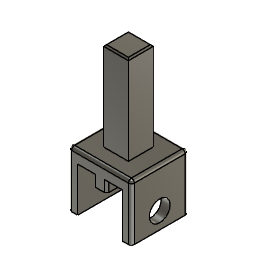
Slider (Autodesk Fusion 360 design; units mm, degrees)
Autodesk Fusion 360 part; units mm, degrees
sketch "Sketch1" plane through (0, 0, 0) normal (0, 1, 0) x (1, 0, 0)
  line L0 (0, 0) -> (6, 0)
  line L1 (6, 0) -> (6, -38)
  line L2 (6, -38) -> (0, -38)
  line L3 (0, -38) -> (0, 0)
  line L4 (0, -38) -> (42.4, -38)
  line L5 (42.4, -38) -> (42.4, -30)
  line L6 (42.4, -30) -> (0, -30)
  line L7 (0, -30) -> (0, -38)
  line L8 (42.4, -38) -> (36.4, -38)
  line L9 (36.4, -38) -> (36.4, 0)
  line L10 (36.4, 0) -> (42.4, 0)
  line L11 (42.4, 0) -> (42.4, -38)
  line L12 (16.75, -38) -> (25.65, -38)
  line L13 (25.65, -38) -> (25.65, -22.4)
  line L14 (25.65, -22.4) -> (16.75, -22.4)
  line L15 (16.75, -22.4) -> (16.75, -38)
  dimension "d1" = 6
  dimension "d2" = 38
  dimension "d3" = 8
  dimension "d5" = 6
  dimension "d6" = 38
  dimension "d8" = 15.6
  dimension "d9" = 10.75
  dimension "d29" = 10.75
  dimension "d30" = 42.4
  constraint horizontal L0
  constraint vertical L1
  constraint horizontal L2
  constraint vertical L3
  constraint coincident L0.start L3.end
  constraint horizontal L4
  constraint vertical L5
  constraint horizontal L6
  constraint vertical L7
  constraint horizontal L8
  constraint vertical L9
  constraint horizontal L10
  constraint vertical L11
  constraint horizontal L12
  constraint vertical L13
  constraint horizontal L14
  constraint vertical L15
  constraint coincident L4 L12.start
  measures "d1" distance of L0.start L0.end
  measures "d2" distance of L0.start L2.end
  measures "d3" distance of L2.end L6.end
  measures "d5" distance of L4.end L8.end
  measures "d6" distance of L4.end L10.end
  measures "d8" distance of L12.start L14.end L0.start
  measures "d9" distance of L1 L15 L0.start
  measures "d29" distance of L9 L13
  measures "d30" distance of L3 L11
extrude "Extrude1" add sketch "Sketch1" along normal blind 38.4
sketch "Sketch2" plane through (0, 0, 38) normal (0, 0, 1) x (-1, 0, 0)
  line L0 (0, 0) -> (-42.4, 0)
  line L1 (-42.4, 0) -> (-42.4, -38.4)
  line L2 (-42.4, -38.4) -> (0, -38.4)
  line L3 (0, -38.4) -> (0, 0)
  line L4 (-42.4, -38.4) -> (0, 0) construction
  line L5 (0, -38.4) -> (-42.4, 0) construction
  line L6 (-29.6, -10.8) -> (-12.8, -10.8)
  line L7 (-12.8, -10.8) -> (-12.8, -27.6)
  line L8 (-12.8, -27.6) -> (-29.6, -27.6)
  line L9 (-29.6, -27.6) -> (-29.6, -10.8)
  line L10 (-29.6, -10.8) -> (-12.8, -27.6) construction
  line L11 (-12.8, -10.8) -> (-29.6, -27.6) construction
  point P0 (-21.2, -19.2)
  dimension "d12" = 16.8
  dimension "d13" = 16.8
  constraint coincident L1.end L2.start
  constraint coincident L0.start L3.end
  constraint coincident L2.end L3.start
  constraint coincident L0.end L1.start
  constraint perpendicular L6 L7
  constraint parallel L6 L8
  constraint parallel L7 L9
  constraint horizontal L6
  constraint coincident L10 P0
  constraint coincident L11 P0
  constraint midpoint L4 P0
  measures "d12" distance of L6.end L7.end
  measures "d13" distance of L7.end L8.end
extrude "Extrude2" add sketch "Sketch2" along normal blind 60 contours L6 L7 L8 L9
chamfer "Chamfer1" distance 1 angle 45 4 edges at (21.2, 10.8, 98) (29.6, 19.2, 98) (12.8, 19.2, 98) (21.2, 27.6, 98)
sketch "Sketch3" plane through (0, 0, 0) normal (-1, 0, 0) x (0, -1, 0)
  line L0 (0, 0) -> (0, 38)
  line L1 (0, 38) -> (-38.4, 38)
  line L2 (-38.4, 38) -> (-38.4, 0)
  line L3 (-38.4, 0) -> (0, 0)
  line L4 (-38.4, 0) -> (0, 0)
  line L5 (0, 0) -> (0, 22.4)
  line L6 (0, 22.4) -> (-38.4, 22.4)
  line L7 (-38.4, 22.4) -> (-38.4, 0)
  line L8 (-38.4, 22.4) -> (0, 0) construction
  line L9 (0, 22.4) -> (-38.4, 0) construction
  circle A0 centre (-19.2, 11.2) radius 6
  dimension "d18" = 22.4
  dimension "d19" = 12
  constraint horizontal L4
  constraint vertical L5
  constraint horizontal L6
  constraint vertical L7
  constraint coincident L2.end L3.start
  constraint midpoint L9 A0.centre
  measures "d18" distance of L2.end L6.end
  measures "d19" diameter of A0
extrude "Extrude3" cut sketch "Sketch3" against normal up to surface (6 mm away) contours A0
sketch "Sketch4" plane through (42.4, 0, 0) normal (1, 0, 0) x (0, 1, 0)
  line L0 (0, 38) -> (0, 0)
  line L1 (0, 0) -> (38.4, 0)
  line L2 (38.4, 0) -> (38.4, 38)
  line L3 (38.4, 38) -> (0, 38)
  circle A0 centre (19.2, 11.2) radius 6
  circle A1 centre (19.2, 11.2) radius 7
  dimension "d22" = 1
extrude "Extrude4" cut sketch "Sketch4" against normal up to surface (6 mm away) contours A0 | A1
thread "Thread1" "ISO Metric profile 12.0 M12x1.75 6H" major diameter 12.2265 minor diameter 10.2735 pitch 1.75 angle 60 modelled right hand crest width 0.4769 on face at (4, 13.2075, 10.9009) crest through (0.4375, 14.0633, 11.2)
fillet "Fillet1" radius 2 8 edges at (21.2, 0, 38) (0, 19.2, 38) (21.2, 38.4, 38) (42.4, 19.2, 38) (42.4, 38.4, 19) (42.4, 0, 19) (0, 0, 19) (0, 38.4, 19)
chamfer "Chamfer2" distance 1.5 angle 45 4 edges at (16.75, 0, 26.2) (25.65, 0, 26.2) (16.75, 38.4, 26.2) (25.65, 38.4, 26.2)
equation "d8 = 8 mm + 7.6 mm"
equation "d30 = 38.40 mm + 2 mm + 2 mm"
